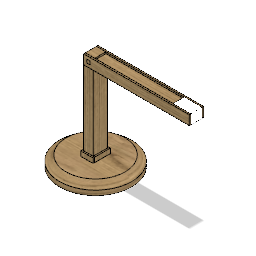
03-Wooden Lamp v2 (Autodesk Fusion 360 design; units mm, degrees)
Autodesk Fusion 360 part; units mm, degrees
note: some values were not read from the file. Chosen so that the rebuilt part matches the saved one: which bodies a step acts on; which face or edge a step refers to.
sketch "Sketch1" plane through (0, 0, 0) normal (0, 0, 1) x (1, 0, 0)
  line L0 (-75, 0) -> (0, 0)
  line L1 (0, 10) -> (-75, 10)
  line L2 (-75, 10) -> (-75, 0)
  line L3 (-75, 10) -> (-61.3538, 20.5454)
  line L4 (-61.3538, 20.5454) -> (0, 20.5454)
  line L5 (0, 0) -> (0, 20.5454)
  constraint horizontal L0
  constraint horizontal L1
  constraint vertical L2
  constraint perpendicular L2 L4
  constraint coincident L0.end L5.start
  constraint perpendicular L4 L5
  constraint coincident L5 L1.start
revolve "Revolve1" add sketch "Sketch1" angle 360 about axis through (0, 1.75, 0) along (0, 1, 0) makes body 1
sketch "Sketch2" plane through (0, 0, 0) normal (0, -1, 0) x (1, 0, 0)
  circle A0 centre (0, 0) radius 75
  line L0 (11.6917, -21.922) -> (-20, 37.5) construction
  line L1 (20, 37.5) -> (-20, -37.5) construction
  line L2 (-15, -22.5) -> (-15, 37.5)
  line L3 (-15, 37.5) -> (-45, 37.5)
  line L4 (-45, 37.5) -> (-45, -22.5)
  line L5 (-45, -22.5) -> (-15, -22.5)
  dimension "d8" = 30
  constraint coincident L0 A0.centre
  constraint coincident L1 A0.centre
  constraint coincident A0.centre origin
  constraint perpendicular L2 L3
  constraint parallel L2 L4
  constraint parallel L3 L5
  measures "d8" distance of L3.end L2.end
extrude "Extrude1" cut sketch "Sketch2" against normal blind 15 contours L2 L3 L4 L5 bodies 1
sketch "Sketch3" plane through (0, 20.5454, 0) normal (0, 1, 0) x (-1, 0, 0)
  circle A0 centre (0, 0) radius 61.3538
  line L0 (10, -15) -> (-10, -15)
  line L1 (-10, -15) -> (-10, 15)
  line L2 (-10, 15) -> (10, 15)
  line L3 (10, 15) -> (10, -15)
  constraint horizontal L0
  constraint vertical L1
  constraint horizontal L2
  constraint vertical L3
extrude "Extrude2" add sketch "Sketch3" along normal blind 200 separate body contours L0 L1 L2 L3 makes body 2
extrude "Extrude3" cut 1 faces at (-3.3333, 20.5454, -5) along direction (0, -1, 0) blind 15 on bodies 2 bodies 1
sketch "Sketch5" plane through (0, 20.5454, 0) normal (0, 1, 0) x (-1, 0, 0)
  line L0 (-10, -15) -> (-10, 15)
  line L1 (-10, 15) -> (10, 15)
  line L2 (10, 15) -> (10, -15)
  line L3 (10, -15) -> (-10, -15)
  circle A0 centre (0, 0) radius 61.3538
  line L4 (-13, 18) -> (13, 18)
  line L5 (13, 18) -> (13, -18)
  line L6 (13, -18) -> (-13, -18)
  line L7 (-13, -18) -> (-13, 18)
  dimension "d12" = -3
extrude "Extrude4" add sketch "Sketch5" along normal blind 10 contours L4 L5 L6 L7 bodies 1
move_body "Move1" bodies 2 to x (1, 0, 0) y (0, 1, 0) z (0, 0, 1) at (0, 40, 0)
move_body "Align1" bodies 2 to x (1, 0, 0) y (0, 1, 0) z (0, 0, 1) at (0, -55, 0)
sketch "Sketch6" plane through (0, 0, 18) normal (0, 0, 1) x (1, 0, 0)
  line L0 (-13, 20.5454) -> (13, 20.5454)
  line L1 (13, 20.5454) -> (13, 30.5454)
  line L2 (13, 30.5454) -> (-13, 30.5454)
  line L3 (-13, 30.5454) -> (-13, 20.5454)
  line L4 (-5, 27) -> (5, 27)
  line L5 (5, 27) -> (5, 23)
  line L6 (5, 23) -> (-5, 23)
  line L7 (-5, 23) -> (-5, 27)
  line L8 (-5, 27) -> (5, 23) construction
  line L9 (5, 27) -> (-5, 23) construction
  point P0 (0, 25)
  constraint horizontal L4
  constraint perpendicular L4 L5
  constraint parallel L4 L6
  constraint parallel L5 L7
  constraint coincident L8 P0
  constraint coincident L9 P0
extrude "Extrude5" cut sketch "Sketch6" against normal blind 36 contours L4 L5 L6 L7 bodies 1 2
extrude "Extrude6" add sketch "Sketch6" against normal blind 36 separate body contours L4 L5 L6 L7 makes body 3
split "Split1" by plane through (0, 20.5454, 0) normal (0, 1, 0) bodies 1 makes body 4 at (13, 23.8787, -6)
split "Split2" by plane through (10, 20.5454, 15) normal (0, 0, -1) bodies 4 makes body 5 at (13, 23.8787, -7)
combine "Combine1" operation add target body 1 tool bodies 5
combine "Combine2" operation add target body 4 tool bodies 3
scale "Scale1" factor 1.5 about (5, 27, 15) bodies 2 1 4
extrude "Extrude7" add 1 faces at (-55, 9, 18.75) along direction (0, -1, 0) blind 2.5 on bodies 1 bodies 1
sketch "Sketch7" plane through (12.5, 0, 0) normal (1, 0, 0) x (0, 0, -1)
  line L0 (-15, -5.1819) -> (30, -5.1819)
  line L1 (30, -5.1819) -> (30, 294.8181)
  line L2 (30, 294.8181) -> (-15, 294.8181)
  line L3 (-15, 294.8181) -> (-15, -5.1819)
  line L4 (30, 294.8181) -> (-15, 294.8181)
  line L5 (-15, 294.8181) -> (-15, 264.8181)
  line L6 (-15, 264.8181) -> (30, 264.8181)
  line L7 (30, 264.8181) -> (30, 294.8181)
  line L8 (-10, 269.8181) -> (25, 269.8181)
  line L9 (25, 269.8181) -> (25, 289.8181)
  line L10 (25, 289.8181) -> (-10, 289.8181)
  line L11 (-10, 289.8181) -> (-10, 269.8181)
  line L12 (-10, 289.8181) -> (-10, 294.8181)
  line L13 (-10, 269.8181) -> (-10, 264.8181)
  line L14 (25, 294.8181) -> (25, 289.8181)
  line L15 (25, 269.8181) -> (25, 264.8181)
  line L16 (-10, 269.8181) -> (-15, 269.8181)
  line L17 (25, 269.8181) -> (30, 269.8181)
  dimension "d22" = 30
  dimension "d23" = -5
  constraint horizontal L4
  constraint vertical L5
  constraint horizontal L6
  constraint vertical L7
  constraint coincident L1.end L2.start
  constraint perpendicular L4 L12
  constraint coincident L2 L12.end
  constraint perpendicular L6 L13
  constraint coincident L6 L13.end
  constraint coincident L2 L14.start
  constraint perpendicular L10 L14
  constraint coincident L6 L15.end
  constraint perpendicular L6 L15
  constraint perpendicular L3 L16
  constraint perpendicular L9 L17
  constraint coincident L3 L16.end
  constraint coincident L1 L17.end
  measures "d22" distance of L1.end L6.end
extrude "Extrude11" add sketch "Sketch7" along normal blind 300 separate body contours L3 L5 L6 L13 L16 | L1 L6 L7 L15 L17 | L2 L3 L4 L5 L11 L12 L16 | L1 L2 L4 L7 L9 L14 L17 | L8 L9 L10 L11 makes body 6
extrude "Extrude12" cut sketch "Sketch7" against normal blind 30 contours L3 L5 L6 L13 L16 | L1 L6 L7 L15 L17 | L2 L3 L4 L5 L11 L12 L16 | L1 L2 L4 L7 L9 L14 L17 bodies 2
extrude "Extrude13" add sketch "Sketch7" against normal blind 30 contours L3 L5 L6 L13 L16 | L1 L6 L7 L15 L17 | L2 L3 L4 L5 L11 L12 L16 | L1 L2 L4 L7 L9 L14 L17 bodies 6
sketch "Sketch8" plane through (0, 0, 15) normal (0, 0, 1) x (1, 0, 0)
  line L0 (-17.5, 264.8181) -> (312.5, 264.8181)
  line L1 (312.5, 264.8181) -> (312.5, 294.8181)
  line L2 (312.5, 294.8181) -> (-17.5, 294.8181)
  line L3 (-17.5, 294.8181) -> (-17.5, 264.8181)
  line L4 (302.5, 274.8181) -> (302.5, 284.8181)
  line L5 (2.5, 284.8181) -> (-7.5, 284.8181)
  line L6 (-7.5, 284.8181) -> (-7.5, 274.8181)
  line L7 (-7.5, 274.8181) -> (2.5, 274.8181)
  line L8 (12.5, -5.1819) -> (12.5, 264.8181)
  line L9 (2.5, 274.8181) -> (2.5, 284.8181)
  constraint parallel L1 L4
  constraint parallel L2 L5
  constraint parallel L3 L6
  constraint parallel L0 L7
extrude "Extrude14" cut sketch "Sketch8" against normal blind 45 contours L5 L6 L7 L9 bodies 2 6
shell "Shell1" thickness 5 removed faces 1 at (-7.5, -5.1819, -15) on bodies 2
extrude "Extrude15" cut 1 faces at (-5.8333, 16, -13.3333) along direction (0, 1, 0) blind 268.8181 on bodies 2 bodies 2 4 makes body 7 at (-5, 27, -28.1667)
shell "Shell2" thickness 5 removed faces 1 at (12.5, 276.4847, -1.6667) on bodies 6
extrude "Extrude16" add sketch "Sketch8" against normal blind 45 separate body contours L5 L6 L7 L9 makes body 8
extrude "Extrude17" add sketch "Sketch7" along normal blind 45 from surface at 250 separate body contours L6 L8 L13 L15 makes body 9
extrude "Extrude18" add 1 faces at (307.5, 268.1514, -1.6667) along direction (1, 0, 0) blind 5 on bodies 9 bodies 9
copy_body "CopyPasteBodies1" bodies 9 makes body 10
move_body "Move2" bodies 10 to x (1, 0, 0) y (0, 1, 0) z (0, 0, 1) at (0, 25, 0)
sketch "Sketch9" plane through (312.5, 0, 0) normal (1, 0, 0) x (0, 0, -1)
  line L0 (-10, 294.8181) -> (-10, 289.8181)
  line L1 (-10, 289.8181) -> (25, 289.8181)
  line L2 (25, 289.8181) -> (25, 294.8181)
  line L3 (25, 294.8181) -> (-10, 294.8181)
  line L4 (-10, 294.8181) -> (25, 294.8181)
  line L5 (25, 294.8181) -> (25, 265)
  line L6 (25, 265) -> (-10, 265)
  line L7 (-10, 265) -> (-10, 294.8181)
  constraint horizontal L4
  constraint vertical L5
  constraint horizontal L6
  constraint vertical L7
  constraint coincident L0.start L3.end
extrude "Extrude19" add sketch "Sketch9" along normal blind 5 bodies 9 10
sketch "Sketch10" plane through (312.5, 0, 0) normal (1, 0, 0) x (0, 0, -1)
  line L0 (-10, 269.8181) -> (25, 269.8181)
  line L1 (25, 269.8181) -> (25, 264.8181)
  line L2 (25, 264.8181) -> (30, 264.8181)
  line L3 (30, 264.8181) -> (30, 294.8181)
  line L4 (30, 294.8181) -> (25, 294.8181)
  line L5 (25, 294.8181) -> (25, 289.8181)
  line L6 (25, 289.8181) -> (-10, 289.8181)
  line L7 (-10, 289.8181) -> (-10, 294.8181)
  line L8 (-10, 294.8181) -> (-15, 294.8181)
  line L9 (-15, 294.8181) -> (-15, 264.8181)
  line L10 (-15, 264.8181) -> (-10, 264.8181)
  line L11 (-10, 264.8181) -> (-10, 269.8181)
  line L12 (-10, 289.8181) -> (-10, 269.8181)
  line L13 (25, 289.8181) -> (25, 269.8181)
  line L14 (25, 269.8181) -> (-10, 269.8181)
  line L15 (-10, 289.8181) -> (25, 289.8181)
  constraint coincident L6.end L7.start
  constraint coincident L0.start L11.end
  constraint coincident L5.end L6.start
  constraint coincident L0.end L1.start
extrude "Extrude20" cut sketch "Sketch10" against normal blind 5 contours L0 L6 L12 L13 L14 L15 bodies 6
move_body "Move3" bodies 9 to x (1, 0, 0) y (0, 1, 0) z (0, 0, 1) at (-5, 0, 0)
sketch "Sketch11" plane through (307.5, 0, 0) normal (-1, 0, 0) x (0, 0, 1)
  line L0 (-25, 269.8181) -> (10, 269.8181)
  line L1 (10, 269.8181) -> (10, 289.8181)
  line L2 (10, 289.8181) -> (-25, 289.8181)
  line L3 (-25, 289.8181) -> (-25, 269.8181)
  line L4 (-25, 284.8181) -> (10, 284.8181)
  line L5 (10, 284.8181) -> (-25, 284.8181)
  line L6 (-25, 274.8181) -> (10, 274.8181)
  line L7 (10, 274.8181) -> (-25, 274.8181)
extrude "Extrude21" add sketch "Sketch11" along normal blind 10 contours L1 L3 L4 L5 L6 L7 bodies 9
extrude "Extrude22" add 1 faces at (297.5, 281.4847, -13.3333) along direction (-1, 0, 0) blind 15 on bodies 9 bodies 9
sketch "Sketch12" plane through (-25, 0, 0) normal (-1, 0, 0) x (0, 0, 1)
  line L0 (48.75, 6.5) -> (-41.25, 6.5)
  line L1 (-41.25, 6.5) -> (-41.25, -13.5)
  line L2 (-41.25, -13.5) -> (48.75, -13.5)
  line L3 (48.75, -13.5) -> (48.75, 6.5)
  line L4 (10, -5.1819) -> (-25, -5.1819)
  line L5 (-25, -5.1819) -> (-25, 6.5)
  line L6 (-25, 6.5) -> (10, 6.5)
  line L7 (10, 6.5) -> (10, -5.1819)
  constraint coincident L4.end L5.start
  constraint coincident L0 L5.end
  constraint perpendicular L0 L5
  constraint coincident L0 L6.end
  constraint coincident L4.start L7.end
  constraint perpendicular L4 L7
extrude "Extrude23" cut sketch "Sketch12" against normal blind 15 contours L0 L4 L5 L6 L7 bodies 1
extrude "Extrude24" add 1 faces at (257.5, 268.1514, -1.6667) along direction (-1, 0, 0) blind 50 on bodies 9 bodies 9
